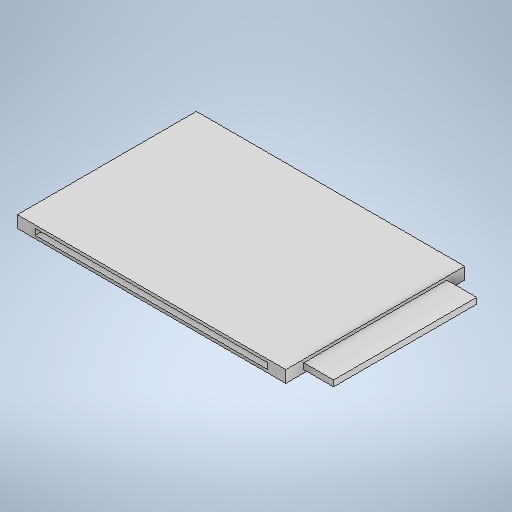
# Autodesk Inventor part: TSU_FM_Floor
Saved by Autodesk Inventor 2025.2 (Build 292293000, 293)
## iProperties
Created: 2025-01-07
Part Number: TSU_FM_Floor
Material: Generic
Document SubType Name: Modeling
Designer: Matt Tidd
Density: 1 g/cm^3
Appearance: Default
Author: Matt Tidd
Autodesk Inventor part; units mm, degrees
ref_plane "YZ Plane" through (0, 0, 0) normal (1, 0, 0) x (0, 1, 0)
ref_plane "XZ Plane" through (0, 0, 0) normal (0, 1, 0) x (-1, 0, 0)
ref_plane "XY Plane" through (0, 0, 0) normal (0, 0, 1) x (1, 0, 0)
sketch "Sketch1" plane through (0, 0, 0) normal (0, 1, 0) x (-1, 0, 0)
  line L0 (0, 0) -> (225, 0)
  line L1 (225, 0) -> (225, -150)
  line L2 (225, -150) -> (0, -150)
  line L3 (0, -150) -> (0, 0)
  dimension "d0" = 225
  dimension "d1" = 150
  constraints: 8 end point, 2 parallel, 1 horizontal, 1 perpendicular
  measures "d0" distance of L1.end L2.end
  measures "d1" distance of L0.end L1.end
extrude "Extrusion1" add sketch "Sketch1" along normal blind 10
sketch "Sketch2" plane through (0, 0, 0) normal (1, 0, 0) x (0, 0, -1)
  line L0 (0, 7.5) -> (150, 7.5)
  line L1 (150, 7.5) -> (150, 2.5)
  line L2 (150, 2.5) -> (0, 2.5)
  line L3 (0, 2.5) -> (0, 7.5)
  line L4 (150, 7.5) -> (135, 7.5)
  line L5 (135, 7.5) -> (135, 1.8795)
  line L6 (135, 1.8795) -> (150, 1.8795)
  line L7 (150, 1.8795) -> (150, 7.5)
  line L8 (0, 2.5) -> (15, 2.5)
  line L9 (15, 2.5) -> (15, 7.5)
  line L10 (15, 7.5) -> (0, 7.5)
  line L11 (0, 7.5) -> (0, 2.5)
  point P0 (0, 0)
  point P1 (135, 2.5)
  dimension "d4" = 150
  dimension "d5" = 5
  dimension "d6" = 15
  dimension "d7" = 15
  constraints: 24 end point, 6 parallel, 3 horizontal, 3 perpendicular, 1 point on line
  measures "d4" distance of L1.end L2.end
  measures "d5" distance of L0.end L1.end
  measures "d6" distance of L6.end L5.end
  measures "d7" distance of L10.end L9.end
sketch "Sketch3" plane through (-225, 0, 0) normal (0, 0, 1) x (1, 0, 0)
  line L0 (0, 7.5) -> (225, 7.5)
  line L1 (225, 7.5) -> (225, 2.5)
  line L2 (225, 2.5) -> (0, 2.5)
  line L3 (0, 2.5) -> (0, 7.5)
  line L4 (225, 7.5) -> (210, 7.5)
  line L5 (210, 7.5) -> (210, 2.5)
  line L6 (210, 2.5) -> (225, 2.5)
  line L7 (225, 2.5) -> (225, 7.5)
  line L8 (0, 7.5) -> (15, 7.5)
  line L9 (15, 7.5) -> (15, 2.5)
  line L10 (15, 2.5) -> (0, 2.5)
  line L11 (0, 2.5) -> (0, 7.5)
  point P0 (225, 0)
  dimension "d8" = 5
  dimension "d9" = 15
  dimension "d10" = 5
  dimension "d11" = 15
  dimension "d12" = 5
  constraints: 24 end point, 6 parallel, 3 horizontal, 3 perpendicular
  measures "d8" distance of L0.end L1.end
  measures "d9" distance of L6.end L5.end
  measures "d10" distance of L5.end L4.end
  measures "d11" distance of L9.end L10.end
  measures "d12" distance of L8.end L9.end
extrude "Extrusion2" cut sketch "Sketch3" against normal blind 25 contours L0 L5 L2 L9
extrude "Extrusion3" add sketch "Sketch2" along normal blind 25 contours L0 L5 L2 L9
body "Solid1"
